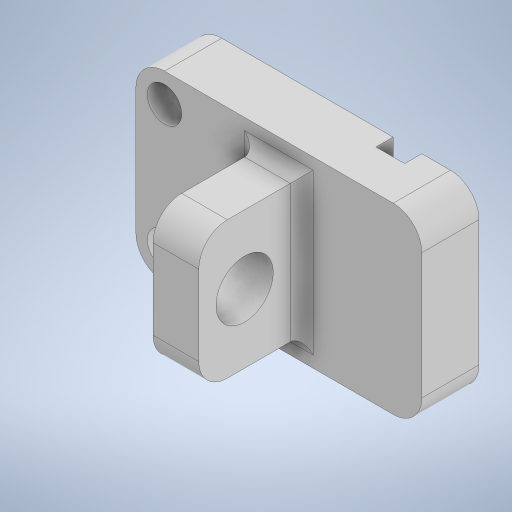
# Autodesk Inventor part: Bartosz_Zukowski_IP_model_4.ipj
Saved by Autodesk Inventor 2024 (Build 280153000, 153)
## iProperties
Created: 2024-03-18
Part Number: Bartosz_Zukowski_IP_model_4.ipj
Material: Ogólny
Document SubType Name: Modeling
Designer: Bartosz
Density: 1 g/cm^3
Appearance: Domyślna
Author: Bartosz
Autodesk Inventor part; units mm, degrees
ref_plane "YZ Plane" through (0, 0, 0) normal (1, 0, 0) x (0, 1, 0)
ref_plane "XZ Plane" through (0, 0, 0) normal (0, 1, 0) x (-1, 0, 0)
ref_plane "XY Plane" through (0, 0, 0) normal (0, 0, 1) x (1, 0, 0)
sketch "Szkic1" plane through (0, 0, 0) normal (0, 0, 1) x (1, 0, 0)
  line L0 (-20, 16) -> (20, 16)
  line L1 (25, 11) -> (25, -11)
  line L2 (20, -16) -> (-20, -16)
  line L3 (-25, -11) -> (-25, 11)
  line L4 (-25, 16) -> (25, -16) construction
  line L5 (25, 16) -> (-25, -16) construction
  arc A0 (25, 11) -> (20, 16) centre (20, 11) ccw
  arc A1 (20, -16) -> (25, -11) centre (20, -11) ccw
  arc A2 (-25, -11) -> (-20, -16) centre (-20, -11) ccw
  arc A3 (-20, 16) -> (-25, 11) centre (-20, 11) ccw
  circle A4 centre (-20, 11) radius 3
  circle A5 centre (-20, -11) radius 3
  point P0 (0, 0)
  dimension "d0" = 50
  dimension "d1" = 32
  dimension "d3" = 5
  dimension "d4" = 5
  dimension "d5" = 6
  dimension "d6" = 6
  constraints: 12 end point, 8 point on circle, 8 point on line, 8 tangent, 6 centre point, 2 coincident, 2 equal radius, 2 midpoint, 2 parallel, 1 horizontal, 1 perpendicular
  measures "d0" distance of L4.end L5.end
  measures "d1" distance of L5.start L4.end
  measures "d3" radius of A0
  measures "d4" radius of A3
  measures "d5" diameter of A4
  measures "d6" diameter of A5
extrude "Wyciągnięcie proste1" add sketch "Szkic1" along normal blind 10
sketch "Szkic2" plane through (0, 0, 10) normal (0, 0, 1) x (1, 0, 0)
  line L0 (-4, -12) -> (4, -12)
  line L1 (4, -12) -> (4, 12)
  line L2 (4, 12) -> (-4, 12)
  line L3 (-4, 12) -> (-4, -12)
  line L4 (-4, -12) -> (4, 12) construction
  line L5 (4, -12) -> (-4, 12) construction
  point P0 (0, 0)
  dimension "d9" = 8
  dimension "d10" = 24
  constraints: 12 end point, 2 midpoint, 2 parallel, 1 horizontal, 1 perpendicular
  measures "d9" distance of L1.end L2.end
  measures "d10" distance of L0.end L1.end
extrude "Wyciągnięcie proste2" add sketch "Szkic2" along normal blind 18
sketch "Szkic3" plane through (4, -12, 10) normal (1, 0, 0) x (0, 0, -1)
  line L0 (0, 24) -> (-18, 24) construction
  line L1 (-9, 24) -> (-9, 0) construction
  line L2 (0, 0) -> (-18, 0) construction
  line L3 (-18, 0) -> (-18, 24) construction
  line L4 (-18, 12) -> (0, 12) construction
  line L5 (0, 23) -> (0, 1) construction
  circle A0 centre (-10, 12) radius 5
  line L6 (-18, 12) -> (-10, 12) construction
  point P0 (10, 12)
  dimension "d13" = 10
  dimension "d28" = 8
  constraints: 6 end point, 4 midpoint, 1 centre point, 1 point on line
  measures "d13" diameter of A0
  measures "d28" distance of L4.start L6.end
extrude "Wyciągnięcie proste3" cut sketch "Szkic3" against normal up to next
fillet "Zaokrąglenie1" radius 2 4 edges at (0, 12, 10) (4, 0, 10) (0, -12, 10) (-4, 0, 10)
fillet "Zaokrąglenie2" radius 5 2 edges at (0, -12, 28) (0, 12, 28)
sketch "Szkic4" plane through (-20, -16, 0) normal (0, -1, 0) x (1, 0, 0)
  line L0 (40, 0) -> (40, 10) construction
  line L1 (45, 0) -> (40, 0) projected
  line L2 (45, 0) -> (35, 0)
  line L3 (35, 0) -> (30, 0)
  line L4 (30, 0) -> (30, 3)
  line L5 (30, 3) -> (35, 3)
  line L6 (35, 3) -> (35, 0)
  dimension "d23" = 10
  dimension "d24" = 5
  dimension "d25" = 3
  constraints: 10 end point, 2 parallel, 1 collinear, 1 horizontal, 1 perpendicular
  measures "d23" distance of L1.start L2.end
  measures "d24" distance of L4.end L5.end
  measures "d25" distance of L3.end L4.end
extrude "Wyciągnięcie proste4" cut sketch "Szkic4" against normal up to next
